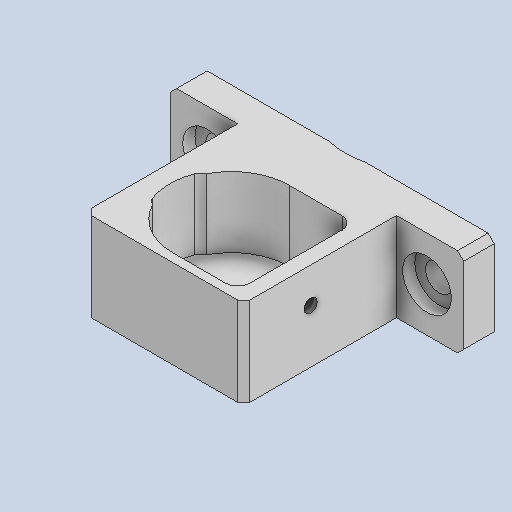
# Autodesk Inventor part: RC04FC-F01-mount-01
Saved by Autodesk Inventor 2024.2 (Build 282272000, 272)
## iProperties
Created: 2021-03-17
Part Number: RC04FC-F01-mount-01
Material: Generic
Document SubType Name: Modeling
Designer: maria
Density: 1 g/cm^3
Appearance: Default
Author: maria
Autodesk Inventor part; units mm, degrees
ref_plane "YZ Plane" through (0, 0, 0) normal (1, 0, 0) x (0, 1, 0)
ref_plane "XZ Plane" through (0, 0, 0) normal (0, 1, 0) x (-1, 0, 0)
ref_plane "XY Plane" through (0, 0, 0) normal (0, 0, 1) x (1, 0, 0)
sketch "Sketch1" plane through (0, 0, 0) normal (0, 0, 1) x (1, 0, 0)
  line L0 (-24, 7.25) -> (24, 7.25)
  line L1 (24, 7.25) -> (24, -7.25)
  line L2 (24, -7.25) -> (-24, -7.25)
  line L3 (-24, -7.25) -> (-24, 7.25)
  point P0 (0, 0)
  dimension "LENGTH" = 48
  dimension "WIDTH" = 14.5
  dimension "d0" = 7.25
  dimension "d3" = 24
  constraints: 8 end point, 2 parallel, 1 horizontal, 1 perpendicular
  measures "LENGTH" distance of L0.start L0.end
  measures "WIDTH" distance of L2.end L0.start
  measures "d0" distance from line of point (0, 0) L0
  measures "d3" distance from line of point (0, 0) L3
extrude "Extrusion1" add sketch "Sketch1" along normal blind 5
sketch "Sketch3" plane through (0, 0, 5) normal (0, 0, 1) x (1, 0, 0)
  line L0 (-24, 7.25) -> (-24, -7.25) projected
  line L1 (24, -7.25) -> (24, 7.25) projected
  point P0 (0, 0)
  point P1 (-18, 0)
  point P2 (18, 0)
  dimension "d13" = 0
  dimension "d14" = 0
  dimension "d15" = 6
  dimension "d16" = 6
  measures "d13" vertical distance of point (18, 0) point (-18, 0)
  measures "d14" vertical distance of point (0, 0) point (18, 0)
  measures "d15" distance from line of L0 point (-18, 0)
  measures "d16" distance from line of L1 point (18, 0)
hole "Hole1" at (-18, 0, 5) at (18, 0, 5) direction (0, 0, -1) diameter 4.5 depth 5 counterbore diameter 8 counterbore depth 2 clearance for "Socket Head Cap Screw" size "#8" standard "Ansi Unified Screw Threads"
sketch "Sketch4" plane through (0, 0, 5) normal (0, 0, 1) x (1, 0, 0)
  line L0 (-13, 7.25) -> (13, 7.25)
  line L1 (13, 7.25) -> (13, -7.25)
  line L2 (13, -7.25) -> (-13, -7.25)
  line L3 (-13, -7.25) -> (-13, 7.25)
  point P0 (0, 0)
  dimension "d17" = 26
  dimension "d18" = 13
  dimension "d19" = 14.5
  dimension "d20" = 7.25
  constraints: 8 end point, 2 parallel, 1 horizontal, 1 perpendicular
  measures "d17" distance of L0.start L0.end
  measures "d18" distance from line of L3 point (0, 0)
  measures "d19" distance of L2.end L0.start
  measures "d20" distance from line of point (0, 0) L0
extrude "Extrusion2" add sketch "Sketch4" along normal blind 25
sketch "Sketch5" plane through (-24, 7.25, 0) normal (0, 1, 0) x (1, 0, 0)
  circle A0 centre (24, -19.05) radius 9.55
  line L0 (14.475, -19.05) -> (33.525, -19.05)
  line L1 (24, -28.6) -> (34.6, -28.6)
  line L2 (34.6, -28.6) -> (34.6, -9.5)
  line L3 (34.6, -9.5) -> (24, -9.5)
  line L4 (24, -9.5) -> (24, -28.6)
  circle A1 centre (24, -19.05) radius 10.05
  circle A2 centre (15.9891, -16.1343) radius 1.525
  circle A3 centre (15.9891, -21.9657) radius 1.525
  line L5 (24, -19.05) -> (15.9891, -16.1343)
  line L6 (15.9891, -21.9657) -> (24, -19.05)
  point P0 (24, 0)
  point P1 (24, -28.6)
  point P2 (24, -9.5)
  point P3 (15.5042, -14.6884)
  point P4 (14.5561, -15.6127)
  point P5 (14.5561, -22.4873)
  point P6 (15.5042, -23.4116)
  dimension "d23" = 0
  dimension "d24" = 19.05
  dimension "DIAMETER" = 19.1
  dimension "d26" = 0
  dimension "d30" = 10.6
  dimension "d31" = 0
  dimension "d32" = 9.55
  dimension "d33" = 9.55
  dimension "d48" = 20.1
  dimension "d49" = 3.05
  dimension "d50" = 3.05
  dimension "d51" = 20
  dimension "d52" = 20
  dimension "d53" = 8.525
  dimension "d54" = 8.525
  constraints: 14 end point, 4 centre point, 2 horizontal, 2 parallel, 1 coincident, 1 perpendicular
  measures "d23" horizontal distance of point (24, 0) A0.centre
  measures "d24" distance of point (24, 0) A0.centre
  measures "DIAMETER" diameter of A0
  measures "d26" distance from line of A0.centre L0
  measures "d30" distance from line of A0.centre L2
  measures "d31" distance from line of A0.centre L4
  measures "d32" distance from line of L1 A0.centre
  measures "d33" distance from line of L3 A0.centre
  measures "d48" diameter of A1
  measures "d49" diameter of A3
  measures "d50" diameter of A2
  measures "d51" angle of L0 L5
  measures "d52" angle of L6 L0
  measures "d53" distance of L5.start L5.end
  measures "d54" distance of L6.start L5.start
extrude "Extrusion3" cut sketch "Sketch5" against normal blind 11.5 contours A0 L4 | A0 L3 A1 L1 | L4 L5 A2 A0 | A0 A3 L6 L4 | A2 A0 | A0 A2 | L3 L2 L1 A1 | L6 A3 A0 A2 L5 | A3 A0 | A0 A3 | A0 A3 A1 A2
fillet "Fillet1" radius 2 2 edges at (10.6, 1.5, 28.6) (10.6, 1.5, 9.5)
sketch "Sketch6" plane through (13, -7.25, 5) normal (1, 0, 0) x (0, 0, -1)
  line L0 (0, 14.5) -> (-25, 14.5) projected
  point P0 (5, 7.25)
  point P1 (-14.05, 8.75)
  dimension "d46" = 19.05
  dimension "d47" = 5.75
  measures "d46" horizontal distance of point (-14.05, 8.75) point (5, 7.25)
  measures "d47" distance from line of L0 point (-14.05, 8.75)
hole "Hole2" at (13, 1.5, 19.05) direction (-1, 0, 0) diameter 2.1565 depth 2.4 thread size "4-40 UNC" class "2B" standard "ANSI Unified Screw Threads"
chamfer "Chamfer1" distance 1 angle 45 6 edges at (13, 0, 30) (-13, 0, 30) (-24, 7.25, 2.5) (-24, -7.25, 2.5) (24, 7.25, 2.5) (24, -7.25, 2.5)
sketch "Sketch7" plane through (0, 0, 0) normal (0, 0, -1) x (-1, 0, 0)
  line L0 (-5.5, 0) -> (-4.5, 0) construction
  line L1 (-5.5, -1.05) -> (-4.5, -1.05)
  line L2 (-4.5, 1.05) -> (-5.5, 1.05)
  arc A0 (-5.5, 1.05) -> (-5.5, -1.05) centre (-5.5, 0) ccw
  arc A1 (-4.5, -1.05) -> (-4.5, 1.05) centre (-4.5, 0) ccw
  point P0 (0, 0)
  point P1 (-5, 0)
  point P2 (5, 0)
  dimension "d58" = 1
  dimension "d59" = 1.05
  dimension "d60" = 10
  dimension "d61" = 0
  dimension "d62" = 0
  dimension "d63" = 5
  constraints: 8 end point, 4 point on circle, 4 tangent, 2 centre point, 1 horizontal, 1 midpoint, 1 parallel
  measures "d58" distance of L0.start L0.end
  measures "d59" radius of A1
  measures "d60" distance of point (-5, 0) point (5, 0)
  measures "d61" vertical distance of point (5, 0) point (-5, 0)
  measures "d62" vertical distance of point (0, 0) point (5, 0)
  measures "d63" distance of point (5, 0) point (0, 0)
hole "Hole3" at (-5, 0, 0) direction (0, 0, 1) diameter 2.1 depth 2.1
extrude "Extrusion4" cut sketch "Sketch7" against normal blind 2.1
sketch "Sketch8" plane through (-23, 7.25, 0) normal (0, 1, 0) x (1, 0, 0)
  circle A0 centre (23, 12.35) radius 12.7
  point P0 (23, 0)
  dimension "d73" = 0
  dimension "d74" = 12.35
  dimension "d75" = 25.4
  constraints: 1 centre point
  measures "d73" horizontal distance of point (23, 0) A0.centre
  measures "d74" distance of point (23, 0) A0.centre
  measures "d75" diameter of A0
extrude "Extrusion5" cut sketch "Sketch8" against normal up to surface (14.5 mm away)
equation "\"d0\" = 0.5 * WIDTH"
equation "\"d3\" = 0.5 * LENGTH"
equation "\"d18\" = 0.5 * d17"
equation "\"d19\" = WIDTH"
equation "\"d20\" = 0.5 * WIDTH"
equation "\"d24\" = BEAM_HEIGHT"
equation "\"d32\" = 0.5 * DIAMETER"
equation "\"d33\" = d32"
equation "\"d54\" = d53"
equation "\"d46\" = BEAM_HEIGHT"
equation "\"d47\" = 0.5 * DEPTH"
equation "\"TOLERANCE\" = 0.1"
equation "\"BEAM_HEIGHT\" = 19.05"
equation "\"DEPTH\" = 11.5"
body "Solid1"
